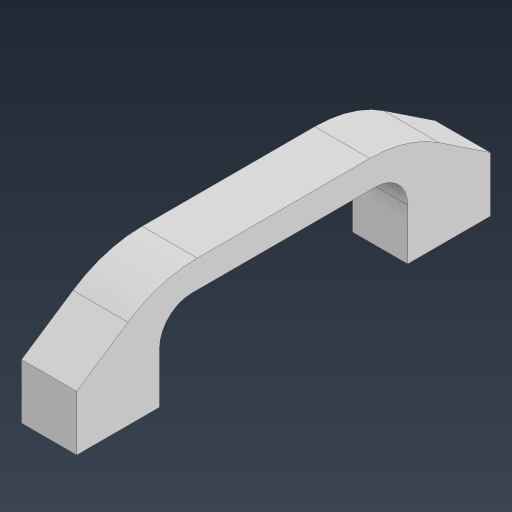
# Autodesk Inventor part: Raczka
Saved by Autodesk Inventor 2024 (Build 280153000, 153)
## iProperties
Created: 2023-12-20
Part Number: Raczka
Material: Generic
Document SubType Name: Modeling
Designer: Piter
Density: 1 g/cm^3
Appearance: Default
Author: Piter
Autodesk Inventor part; units mm, degrees
ref_plane "YZ Plane" through (0, 0, 0) normal (1, 0, 0) x (0, 1, 0)
ref_plane "XZ Plane" through (0, 0, 0) normal (0, 1, 0) x (-1, 0, 0)
ref_plane "XY Plane" through (0, 0, 0) normal (0, 0, 1) x (1, 0, 0)
sketch "Sketch1" plane through (0, 0, 0) normal (1, 0, 0) x (0, 1, 0)
  line L0 (0, 0) -> (0, 45)
  line L1 (0, 45) -> (30, 45)
  line L2 (30, 45) -> (30, -45)
  line L3 (30, -45) -> (0, -45)
  line L4 (0, -45) -> (0, 45)
  line L5 (30, 45) -> (40, 45)
  line L6 (40, 45) -> (40, -45)
  line L7 (40, -45) -> (30, -45)
  line L8 (30, -45) -> (30, 45)
  line L9 (0, 45) -> (20, 45)
  line L10 (20, 45) -> (20, 75)
  line L11 (20, 75) -> (0, 75)
  line L12 (0, 75) -> (0, 45)
  line L13 (30, 0) -> (0, 0)
  line L14 (0, -45) -> (30, -45)
  line L15 (30, -45) -> (40, -45)
  line L16 (0, -45) -> (20, -45)
  line L17 (20, -45) -> (20, -75)
  line L18 (20, -75) -> (0, -75)
  line L19 (0, -75) -> (0, -45)
  line L20 (20, 75) -> (40, 45)
  line L21 (40, -45) -> (20, -75)
  dimension "d0" = 45
  dimension "d1" = 30
  dimension "d2" = 90
  dimension "d3" = 10
  dimension "d4" = 20
  dimension "d5" = 30
  constraints: 44 end point, 6 parallel, 4 perpendicular, 3 horizontal, 3 symmetric about line, 1 midpoint, 1 vertical
  measures "d0" distance of L0.start L0.end
  measures "d1" distance of L2.end L3.end
  measures "d2" distance of L1.end L2.end
  measures "d3" distance of L6.end L7.end
  measures "d4" distance of L11.end L10.end
  measures "d5" distance of L10.end L9.end
extrude "Extrusion1" add sketch "Sketch1" along normal blind 20 contours L12 L11 L10 L1 | L3 L17 L18 L19 | L2 L5 L6 L7 | L10 L20 L5 L1 | L3 L7 L21 L17
sketch "Sketch2" plane through (0, 0, -75) normal (0, -1, 0) x (1, 0, 0)
  line L0 (0, 30) -> (20, 30) projected
  line L1 (10, 30) -> (10, 0)
  line L2 (0, 0) -> (20, 0) projected
  line L3 (10, 30) -> (10, 20)
  line L4 (10, 20) -> (10, 10)
  circle A0 centre (10, 10) radius 3.25
  line L5 (0, 75) -> (24.904, 75)
  circle A1 centre (10, 20) radius 1
  line L6 (10, 130) -> (10, 140)
  circle A2 centre (10, 140) radius 3.25
  circle A3 centre (10, 130) radius 1
  dimension "d8" = 30
  dimension "d9" = 10
  dimension "d10" = 10
  dimension "d11" = 6.5
  dimension "d12" = 2
  constraints: 10 end point, 4 centre point, 4 coincident, 4 symmetric about line, 2 midpoint, 2 point on line, 1 horizontal, 2 other
  measures "d8" distance of L1.start L1.end
  measures "d9" distance of L1.start L3.end
  measures "d10" distance of L3.end L4.end
  measures "d11" diameter of A0
  measures "d12" diameter of A1
extrude "Extrusion2" cut sketch "Sketch2" against normal blind 3.2 contours A0 L1 | L1 A0 | A2
extrude "Extrusion3" cut sketch "Sketch2" against normal blind 10 contours A1 L1 | L1 A1 | A3
fillet "Fillet1" radius 11.5 2 edges at (10, 30, -45) (10, 30, 45)
fillet "Fillet2" radius 45.25 2 edges at (10, 40, -45) (10, 40, 45)
body "Solid1"
